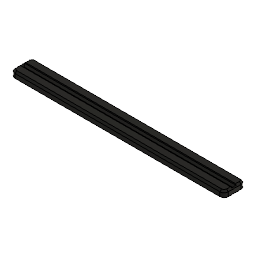
stand (Autodesk Fusion 360 design; units mm, degrees)
Autodesk Fusion 360 part; units mm, degrees
sketch "stand" plane through (0, 0, 0) normal (0, 0, 1) x (1, 0, 0)
  line L0 (-121, 12.5) -> (121, 12.5)
  line L1 (126, 7.5) -> (126, -7.5)
  line L2 (121, -12.5) -> (-121, -12.5)
  line L3 (-126, -7.5) -> (-126, 7.5)
  arc A0 (-121, 12.5) -> (-126, 7.5) centre (-121, 7.5) ccw
  arc A1 (-126, -7.5) -> (-121, -12.5) centre (-121, -7.5) ccw
  arc A2 (121, -12.5) -> (126, -7.5) centre (121, -7.5) ccw
  arc A3 (126, 7.5) -> (121, 12.5) centre (121, 7.5) ccw
  line L4 (0, 1.75) -> (0, 22.5) construction
  line L5 (1.75, 0) -> (22.5, 0) construction
  dimension "d1" = 5
  dimension "d2" = 252
  dimension "d3" = 25
  constraint horizontal L0
  constraint vertical L1
  constraint horizontal L2
  constraint vertical L3
  constraint tangent L3 A0
  constraint tangent L0 A0
  constraint tangent L2 A1
  constraint tangent L3 A1
  constraint equal A0 A1
  constraint tangent L1 A2
  constraint tangent L2 A2
  constraint equal A0 A2
  constraint tangent L0 A3
  constraint tangent L1 A3
  constraint equal A0 A3
  constraint symmetric L1 L3 L4
  constraint symmetric L0 L2 L5
  measures "d1" radius of A0
  measures "d2" distance of L1 L3
  measures "d3" distance of L0 L2
sketch "groove" plane through (0, 0, 0) normal (0, 0, 1) x (1, 0, 0)
  line L0 (-125, 2.55) -> (125, 2.55)
  line L1 (125, 2.55) -> (125, -2.55)
  line L2 (125, -2.55) -> (-125, -2.55)
  line L3 (-125, -2.55) -> (-125, 2.55)
  line L4 (1.75, 0) -> (22.5, 0) construction
  line L5 (0, 1.75) -> (0, 22.5) construction
  dimension "d5" = 5.1
  dimension "d6" = 250
  constraint horizontal L0
  constraint vertical L1
  constraint horizontal L2
  constraint vertical L3
  constraint symmetric L0 L2 L4
  constraint symmetric L1 L3 L5
  measures "d5" distance of L0.start L2.end
  measures "d6" distance of L0.start L0.end
extrude "base (1)" add sketch "stand" against normal blind 7
extrude "groove (1)" cut sketch "groove" against normal blind 5
chamfer "groove chamfer" distance 0.5 angle 60 4 edges at (0, 2.55, 0) (0, -2.55, 0) (-125, 0, 0) (125, 0, 0) measured on face at (40.3333, 5.8667, 0) measured on face at (40.3333, 5.8667, 0) measured on face at (40.3333, 5.8667, 0) measured on face at (40.3333, 5.8667, 0)
chamfer "Chamfer2" distance 2 angle 45 8 edges at (0, -12.5, 0) (-124.5355, -11.0355, 0) (-126, 0, 0) (-124.5355, 11.0355, 0) (0, 12.5, 0) (124.5355, 11.0355, 0) (126, 0, 0) (124.5355, -11.0355, 0) measured on face at (40.3333, -12.5, -2.3333) measured on face at (40.3333, 6.2, 0) measured on face at (-126, -2.5, -2.3333) measured on face at (40.3333, 6.2, 0) measured on face at (-40.3333, 12.5, -2.3333) measured on face at (40.3333, 6.2, 0) measured on face at (126, 2.5, -2.3333) measured on face at (40.3333, 6.2, 0)
named bodies: "Base"
